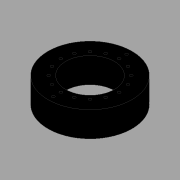
# Autodesk Inventor part: PocketNC_Workpiece_Y_axis_rotation
Saved by Autodesk Inventor 2017 (Build 210142000, 142)
## iProperties
Created: 2018-06-06
Part Number: PocketNC_Workpiece_Y_axis_rotation
Material: Generic
Document SubType Name: Modeling
Designer: Jarrett
Density: 1 g/cm^3
Appearance: Anodized - Black
Author: Jarrett
Autodesk Inventor part; units mm, degrees
ref_plane "YZ Plane" through (0, 0, 0) normal (1, 0, 0) x (0, 1, 0)
ref_plane "XZ Plane" through (0, 0, 0) normal (0, 1, 0) x (-1, 0, 0)
ref_plane "XY Plane" through (0, 0, 0) normal (0, 0, 1) x (1, 0, 0)
sketch "Sketch1" plane through (0, 0, 0) normal (0, 1, 0) x (-1, 0, 0)
  circle A0 centre (0, 0) radius 26
  circle A1 centre (0, 0) radius 44.855
  dimension "d0" = 52
  dimension "d1" = 89.71
  constraints: 2 centre point, 2 coincident
  measures "d0" diameter of A0
  measures "d1" diameter of A1
extrude "Extrusion1" add sketch "Sketch1" along normal blind 27
sketch "Sketch2" plane through (0, 27, 0) normal (0, 1, 0) x (1, 0, 0)
  circle A0 centre (0, 0) radius 26 construction
  line L0 (0, 26) -> (0, 31.1) construction
  circle A1 centre (0, 31.1) radius 1.5
  circle A2 centre (-11.9015, 28.7327) radius 1.5
  circle A3 centre (-21.991, 21.991) radius 1.5
  circle A4 centre (-28.7327, 11.9015) radius 1.5
  circle A5 centre (-31.1, 0) radius 1.5
  circle A6 centre (-28.7327, -11.9015) radius 1.5
  circle A7 centre (-21.991, -21.991) radius 1.5
  circle A8 centre (-11.9015, -28.7327) radius 1.5
  circle A9 centre (0, -31.1) radius 1.5
  circle A10 centre (11.9015, -28.7327) radius 1.5
  circle A11 centre (21.991, -21.991) radius 1.5
  circle A12 centre (28.7327, -11.9015) radius 1.5
  circle A13 centre (31.1, 0) radius 1.5
  circle A14 centre (28.7327, 11.9015) radius 1.5
  circle A15 centre (21.991, 21.991) radius 1.5
  circle A16 centre (11.9015, 28.7327) radius 1.5
  line L1 (0, -31.1) -> (0, -39.25) construction
  circle A17 centre (0, -39.25) radius 1.5
  line L2 (0, 31.1) -> (0, 39.25) construction
  circle A18 centre (0, 39.25) radius 1.5
  dimension "d4" = 5.1
  dimension "d5" = 3
  dimension "d8" = 360
  dimension "d10" = 8.15
  dimension "d11" = 3
  dimension "d12" = 8.15
  dimension "d13" = 3
  constraints: 18 centre point, 6 end point, 3 coincident, 3 vertical, 1 vertical alignment, 34 other
  measures "d4" distance of L0.start L0.end
  measures "d5" diameter of A1
  measures "d10" distance of L1.start L1.end
  measures "d11" diameter of A17
  measures "d12" distance of L2.start L2.end
  measures "d13" diameter of A18
extrude "Extrusion2" cut sketch "Sketch2" against normal blind 12.5
body "Solid1"
